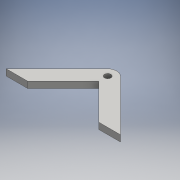
# Autodesk Inventor part: zwo camera support leg
Saved by Autodesk Inventor 2016 (Build 200138000, 138)
## iProperties
Created: 2015-12-13
Part Number: zwo camera support leg
Material: Generic
Document SubType Name: Modeling
Designer: roduino
Density: 1 g/cm^3
Appearance: Default
Author: roduino
Autodesk Inventor part; units mm, degrees
ref_plane "YZ Plane" through (0, 0, 0) normal (1, 0, 0) x (0, 1, 0)
ref_plane "XZ Plane" through (0, 0, 0) normal (0, 1, 0) x (-1, 0, 0)
ref_plane "XY Plane" through (0, 0, 0) normal (0, 0, 1) x (1, 0, 0)
sketch "Sketch1" plane through (0, 0, 0) normal (0, 0, 1) x (1, 0, 0)
  circle A0 centre (0, 35) radius 2.5
  line L0 (-5, 40) -> (-45, 0)
  line L1 (0, 45) -> (5, 40)
  line L2 (0, 45) -> (65, 45) construction
  line L3 (0, 45) -> (0, 0) construction
  arc A1 (5, 40) -> (-5, 40) centre (0, 35) ccw
  line L4 (-27.9289, 0) -> (0, 27.9289)
  line L5 (0, 27.9289) -> (27.9289, 0)
  line L6 (5, 40) -> (45, 0)
  line L7 (-45, 0) -> (-27.9289, 0)
  line L8 (27.9289, 0) -> (45, 0)
  dimension "d0" = 5
  dimension "d1" = 35
  dimension "d4" = 45
  dimension "d5" = 45
  dimension "d6" = 45
  constraints: 18 end point, 3 horizontal, 3 parallel, 2 centre point, 2 point on circle, 2 tangent, 1 coincident, 1 point on line, 1 vertical
  measures "d0" diameter of A0
  measures "d1" distance of L3.end A0.centre
  measures "d4" distance of L3.end L1.start
  measures "d5" angle of L3 L1
  measures "d6" angle of L3 L0
extrude "Extrusion1" add sketch "Sketch1" along normal blind 5
equation "\"d6\" = d5"
body "Solid1"
